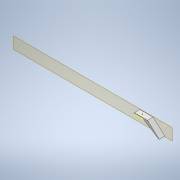
# Autodesk Inventor part: zaślepka-1
Saved by Autodesk Inventor 2022.3 (Build 263350000, 350)
## iProperties
Created: 2022-10-27
Part Number: zaślepka-1
Material: Generic
Document SubType Name: Modeling
Designer: komputer
Density: 1 g/cm^3
Appearance: Default
Author: komputer
Autodesk Inventor part; units mm, degrees
ref_plane "YZ Plane" through (0, 0, 0) normal (1, 0, 0) x (0, 1, 0)
ref_plane "XZ Plane" through (0, 0, 0) normal (0, 1, 0) x (-1, 0, 0)
ref_plane "Work Plane1" through (0, 0, 0) normal (0, 0, 1) x (1, 0, 0)
sketch "Sketch1" plane through (0, 0, 0) normal (0, 0, 1) x (1, 0, 0)
  line L0 (-80.6325, -6) -> (-735.8557, -6) projected
  line L1 (-5.1227, -53.9222) -> (-80.6325, -6) projected
  line L2 (-1.3085, -54) -> (-4.8547, -54) projected
  line L3 (-58.1097, -2) -> (-0.9751, -53.1274) projected
  line L4 (-731.3557, -2) -> (-735.8557, -6) projected
  line L5 (-127.5657, -6) -> (-127.5657, 0)
  arc A0 (-5.1227, -53.9222) -> (-4.8547, -54) centre (-4.8547, -53.5) ccw projected
  arc A1 (-1.3085, -54) -> (-0.9751, -53.1274) centre (-1.3085, -53.5) ccw projected
  line L6 (-58.1097, -2) -> (-731.3557, -2) projected
  point P0 (0, 0)
  point P1 (-127.5657, -2)
  constraints: 2 end point, 1 point on line
ref_plane "Work Plane2" through (-788.7937, -153, 28) normal (0, 0, 1) x (1, 0, 0)
extrude "Extrusion1" add sketch "Sketch1" along normal up to surface (28 mm away) contours L0 L5 L6 L3 A1 L2 A0 L1
sketch "Sketch2" plane through (-127.5657, -6, 0) normal (0, -1, 0) x (1, 0, 0)
  circle A0 centre (27.1635, 14) radius 2.1 projected
  line L0 (27.1635, 14) -> (30.6635, 14)
  line L1 (30.6635, 11.9793) -> (27.1635, 9.9585)
  line L2 (27.1635, 9.9585) -> (23.6635, 11.9793)
  line L3 (23.6635, 11.9793) -> (23.6635, 16.0207)
  line L4 (23.6635, 16.0207) -> (27.1635, 18.0415)
  line L5 (27.1635, 18.0415) -> (30.6635, 16.0207)
  line L6 (30.6635, 16.0207) -> (30.6635, 11.9793)
  point P0 (127.5657, 0)
  dimension "d2" = 3.5
  constraints: 14 end point, 1 coincident, 1 horizontal, 1 midpoint, 13 other
  measures "d2" distance of L0.start L0.end
extrude "Extrusion2" cut sketch "Sketch2" against normal blind 3.6 contours A0 | L6 L1 L2 L3 L4 L5
sketch "Sketch3" plane through (-127.5657, -2.4, 0) normal (0, -1, 0) x (1, 0, 0)
  line L0 (27.1635, 18.0415) -> (30.6635, 16.0207) projected
  line L1 (23.6635, 16.0207) -> (27.1635, 18.0415) projected
  line L2 (23.6635, 11.9793) -> (23.6635, 16.0207) projected
  line L3 (27.1635, 9.9585) -> (23.6635, 11.9793) projected
  line L4 (30.6635, 11.9793) -> (27.1635, 9.9585) projected
  line L5 (30.6635, 16.0207) -> (30.6635, 11.9793) projected
  circle A0 centre (27.1635, 14) radius 2.1
  point P0 (127.5657, 0)
  dimension "d5" = 4.2
  constraints: 1 centre point
  measures "d5" diameter of A0
extrude "Extrusion3" cut sketch "Sketch3" against normal through all contours A0
sketch "Sketch4" plane through (-127.5657, -6, 0) normal (0, -1, 0) x (1, 0, 0)
  line L0 (23.6635, 16.0207) -> (27.1635, 18.0415) projected
  line L1 (27.1635, 18.0415) -> (30.6635, 16.0207) projected
  line L2 (30.6635, 16.0207) -> (30.6635, 11.9793) projected
  line L3 (30.6635, 11.9793) -> (27.1635, 9.9585) projected
  line L4 (27.1635, 9.9585) -> (23.6635, 11.9793) projected
  line L5 (23.6635, 11.9793) -> (23.6635, 16.0207) projected
  line L6 (46.9332, 28) -> (0, 28) projected
  line L7 (0, 0) -> (0, 28) projected
  line L8 (0, 0) -> (46.9332, 0) projected
  line L9 (46.9332, 0) -> (46.9332, 28) projected
  line L10 (49.6735, 14) -> (46.1735, 14)
  line L11 (46.1735, 16.0207) -> (49.6735, 18.0415)
  line L12 (49.6735, 18.0415) -> (53.1735, 16.0207)
  line L13 (53.1735, 16.0207) -> (53.1735, 11.9793)
  line L14 (53.1735, 11.9793) -> (49.6735, 9.9585)
  line L15 (49.6735, 9.9585) -> (46.1735, 11.9793)
  line L16 (46.1735, 11.9793) -> (46.1735, 16.0207)
  circle A0 centre (49.6735, 14) radius 2.1
  line L17 (47.5735, 20) -> (47.5735, 10) projected
  arc A1 (47.5735, 10) -> (51.7735, 10) centre (49.6735, 10) ccw projected
  line L18 (51.7735, 10) -> (51.7735, 20) projected
  arc A2 (51.7735, 20) -> (47.5735, 20) centre (49.6735, 20) ccw projected
  line L19 (45.6735, 10) -> (45.6735, 20) projected
  arc A3 (53.6735, 20) -> (45.6735, 20) centre (49.6735, 20) ccw projected
  line L20 (53.6735, 10) -> (53.6735, 20) projected
  arc A4 (45.6735, 10) -> (53.6735, 10) centre (49.6735, 10) ccw projected
  point P0 (127.5657, 0)
  dimension "d8" = 3.5
  dimension "d9" = 4.2
  constraints: 14 end point, 2 coincident, 1 centre point, 1 horizontal, 1 midpoint, 13 other
  measures "d8" distance of L10.start L10.end
  measures "d9" diameter of A0
extrude "Extrusion4" cut sketch "Sketch4" against normal up to surface (3.6 mm away) contours L11 L17 L10 L9 | L9 L10 L16 L11 | L10 L17 L15 L9 | L9 L15 L16 L10 | L11 L12 L18 A0 L17 | A0 | A0 L18 L14 L15 L17 | L18 L12 L13 L14
sketch "Sketch5" plane through (-127.5657, -6, 0) normal (0, -1, 0) x (1, 0, 0)
  line L0 (46.9332, 11.5407) -> (46.1735, 11.9793) projected
  line L1 (46.1735, 11.9793) -> (46.1735, 16.0207) projected
  line L2 (46.1735, 16.0207) -> (46.9332, 16.4593) projected
  line L3 (46.9332, 16.4593) -> (46.9332, 28) projected
  line L4 (46.9332, 28) -> (0, 28) projected
  line L5 (0, 0) -> (0, 28) projected
  line L6 (0, 0) -> (46.9332, 0) projected
  line L7 (46.9332, 0) -> (46.9332, 11.5407) projected
  line L8 (23.6635, 16.0207) -> (27.1635, 18.0415) projected
  line L9 (27.1635, 18.0415) -> (30.6635, 16.0207) projected
  line L10 (30.6635, 16.0207) -> (30.6635, 11.9793) projected
  line L11 (30.6635, 11.9793) -> (27.1635, 9.9585) projected
  line L12 (27.1635, 9.9585) -> (23.6635, 11.9793) projected
  line L13 (23.6635, 11.9793) -> (23.6635, 16.0207) projected
  line L14 (53.1735, 11.9793) -> (53.1735, 16.0207) projected
  line L15 (49.6735, 9.9585) -> (53.1735, 11.9793) projected
  circle A0 centre (49.6735, 14) radius 2.1 projected
  point P0 (127.5657, 0)
extrude "Extrusion5" cut sketch "Sketch5" along normal blind 10 contours A0
sketch "Sketch6" plane through (-74.3922, -2.4, 11.9793) normal (0, -1, 0) x (1, 0, 0)
  line L0 (-7, 0) -> (-3.5, -2.0207) projected
  line L1 (-3.5, -2.0207) -> (0, 0) projected
  line L2 (0, 0) -> (0, 4.0415) projected
  line L3 (0, 4.0415) -> (-3.5, 6.0622) projected
  line L4 (-3.5, 6.0622) -> (-7, 4.0415) projected
  line L5 (-7, 4.0415) -> (-7, 0) projected
  point P0 (74.3922, -11.9793)
extrude "Extrusion6" cut sketch "Sketch6" along normal blind 10
sketch "Sketch7" plane through (-74.3922, -2.4, 11.9793) normal (0, -1, 0) x (1, 0, 0)
  circle A0 centre (-3.5, 2.0207) radius 2.1 projected
  arc A1 (-3.5, -1.9793) -> (-3.5, 6.0207) centre (-3.5, 2.0207) ccw projected
  line L0 (-26.01, -1.9793) -> (-3.5, -1.9793) projected
  line L1 (-671.6821, 16.0207) -> (3.99, 16.0207) projected
  line L2 (3.99, -58.9793) -> (3.99, 16.0207) projected
  line L3 (-671.6821, -58.9793) -> (3.99, -58.9793) projected
  line L4 (-671.6821, -58.9793) -> (-671.6821, 16.0207) projected
  arc A2 (-30.01, -1.9793) -> (-22.01, -1.9793) centre (-26.01, -1.9793) ccw projected
  line L5 (-22.01, -1.9793) -> (-22.01, 8.0207) projected
  arc A3 (-22.01, 8.0207) -> (-30.01, 8.0207) centre (-26.01, 8.0207) ccw projected
  line L6 (-30.01, 8.0207) -> (-30.01, -1.9793) projected
  arc A4 (-7.5, -1.9793) -> (0.5, -1.9793) centre (-3.5, -1.9793) ccw projected
  line L7 (0.5, -1.9793) -> (0.5, 8.0207) projected
  arc A5 (0.5, 8.0207) -> (-7.5, 8.0207) centre (-3.5, 8.0207) ccw projected
  line L8 (-7.5, 8.0207) -> (-7.5, -1.9793) projected
  point P0 (74.3922, -11.9793)
extrude "Extrusion7" cut sketch "Sketch7" against normal blind 10 contours A0
sketch "Sketch8" plane through (-127.5657, -6, 0) normal (0, -1, 0) x (1, 0, 0)
  line L0 (46.9332, 11.5407) -> (46.1735, 11.9793) projected
  line L1 (46.1735, 11.9793) -> (46.1735, 16.0207) projected
  line L2 (46.1735, 16.0207) -> (46.9332, 16.4593) projected
  line L3 (46.9332, 16.4593) -> (46.9332, 28) projected
  line L4 (46.9332, 28) -> (0, 28) projected
  line L5 (0, 0) -> (0, 28) projected
  line L6 (0, 0) -> (46.9332, 0) projected
  line L7 (46.9332, 0) -> (46.9332, 11.5407) projected
  line L8 (23.6635, 16.0207) -> (27.1635, 18.0415) projected
  line L9 (27.1635, 18.0415) -> (30.6635, 16.0207) projected
  line L10 (30.6635, 16.0207) -> (30.6635, 11.9793) projected
  line L11 (30.6635, 11.9793) -> (27.1635, 9.9585) projected
  line L12 (27.1635, 9.9585) -> (23.6635, 11.9793) projected
  line L13 (23.6635, 11.9793) -> (23.6635, 16.0207) projected
  circle A0 centre (49.6735, 14) radius 5.3947
  line L14 (47.5735, 20) -> (47.5735, 10) projected
  arc A1 (47.5735, 10) -> (51.7735, 10) centre (49.6735, 10) ccw projected
  line L15 (51.7735, 10) -> (51.7735, 20) projected
  arc A2 (51.7735, 20) -> (47.5735, 20) centre (49.6735, 20) ccw projected
  line L16 (45.6735, 10) -> (45.6735, 20) projected
  arc A3 (53.6735, 20) -> (45.6735, 20) centre (49.6735, 20) ccw projected
  line L17 (53.6735, 10) -> (53.6735, 20) projected
  arc A4 (45.6735, 10) -> (53.6735, 10) centre (49.6735, 10) ccw projected
  point P0 (127.5657, 0)
  point P1 (46.9332, 9.3532)
  point P2 (46.9332, 18.6468)
  constraints: 1 centre point
extrude "Extrusion8" cut sketch "Sketch8" along normal blind 10 contours L0 L1 L2 L3 A0 L14 A1 L7 | A1 L14 A0 L15 | A1 L15 A0 L17 | L17 A0
ref_plane "Work Plane3" through (0, -54, -47) normal (-1, 0, 0) x (0, 0, 1)
sketch "Sketch9" plane through (0, -54, -47) normal (-1, 0, 0) x (0, 0, 1)
  line L0 (0, 0.8726) -> (47, 0.8726) projected
  line L1 (0, 63) -> (0, 0.8726) projected
  line L2 (0, 63) -> (75, 63) projected
  line L3 (75, 52) -> (75, 63) projected
  line L4 (47, 52) -> (47, 0.8726) projected
  line L5 (75, 52) -> (75, 0.8726) projected
  line L6 (47, 0.8726) -> (75, 0.8726) projected
  line L7 (47, 0.8726) -> (47, 52) projected
  line L8 (47, 54) -> (75, 54) projected
  line L9 (47, 0.8726) -> (47.3, 0.8726)
  line L10 (47.3, 0.8726) -> (47.3, 54)
  line L11 (47.3, 54) -> (47, 54)
  line L12 (47, 54) -> (47, 0.8726)
  line L13 (47, 52) -> (75, 52) projected
  line L14 (47, 52) -> (75, 52) projected
  dimension "d20" = 0.3
  constraints: 8 end point, 2 parallel, 1 horizontal, 1 perpendicular, 1 point on line
  measures "d20" distance of L11.end L10.end
extrude "Extrusion9" cut sketch "Sketch9" along normal up to surface (127.5657 mm away) contours L4 L13 L10 L6 | L12 L8 L10 L13
body "Solid1"
